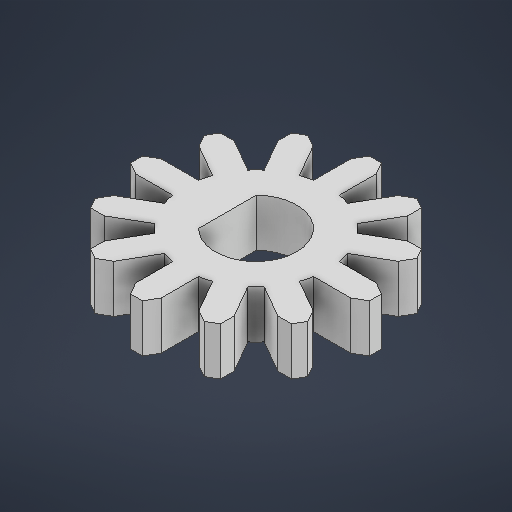
# Autodesk Inventor part: Gear
Saved by Autodesk Inventor 2026.2 (Build 302298010, 298A)
## iProperties
Created: 2026-04-14
Part Number: Gear
Material: Genérico
Document SubType Name: Modeling
Designer: pauli
Density: 1 g/cm^3
Appearance: Padrão
Author: pauli
Autodesk Inventor part; units mm, degrees
ref_plane "YZ Plane" through (0, 0, 0) normal (1, 0, 0) x (0, 1, 0)
ref_plane "XZ Plane" through (0, 0, 0) normal (0, 1, 0) x (-1, 0, 0)
ref_plane "XY Plane" through (0, 0, 0) normal (0, 0, 1) x (1, 0, 0)
sketch "Esboço1" plane through (0, 0, 0) normal (0, 1, 0) x (-1, 0, 0)
  arc A0 (1, 1.118) -> (1, -1.118) centre (0, 0) ccw construction
  line L0 (1, 1.118) -> (1, -1.118) construction
  line L1 (0, 0) -> (-1.5, 0) construction
  line L2 (1.2, -1.2042) -> (1.2, 1.2042)
  arc A1 (1.2, 1.2042) -> (1.2, -1.2042) centre (0, 0) ccw
  circle A2 centre (0, 0) radius 3
  point P0 (1, 0)
  dimension "d0" = 3
  dimension "d1" = 2.5
  dimension "d2" = 0.2
  dimension "d3" = 6
  constraints: 6 end point, 5 point on circle, 3 centre point, 2 coincident, 1 horizontal, 1 midpoint, 1 vertical, 1 other
  measures "d0" diameter of A0
  measures "d1" distance of L1.end point (1, 0)
  measures "d2" distance between parallel lines of L0 L2
  measures "d3" diameter of A2
extrude "Extrusão1" add sketch "Esboço1" along normal blind 2
sketch "Esboço2" plane through (0, 2, 0) normal (0, 1, 0) x (1, 0, 0)
  line L0 (0, 0) -> (-5, 0) construction
  line L1 (-5, 0) -> (-5, 0.25)
  line L2 (-5, 0.25) -> (-4.5, 0.5387)
  line L3 (-4.5, 0.5387) -> (-2.8873, 0.5387)
  line L4 (-5, 0) -> (-5, -0.25)
  line L5 (-5, -0.25) -> (-4.5, -0.5387)
  line L6 (-4.5, -0.5387) -> (-2.8873, -0.5387)
  line L7 (-4.3301, -2.5) -> (-4.4551, -2.2835)
  line L8 (-4.4551, -2.2835) -> (-4.1665, -1.7835)
  line L9 (-4.1665, -1.7835) -> (-2.7698, -0.9771)
  line L10 (-4.3301, -2.5) -> (-4.2051, -2.7165)
  line L11 (-4.2051, -2.7165) -> (-3.6278, -2.7165)
  line L12 (-3.6278, -2.7165) -> (-2.2311, -1.9102)
  line L13 (-2.5, -4.3301) -> (-2.7165, -4.2051)
  line L14 (-2.7165, -4.2051) -> (-2.7165, -3.6278)
  line L15 (-2.7165, -3.6278) -> (-1.9102, -2.2311)
  line L16 (-2.5, -4.3301) -> (-2.2835, -4.4551)
  line L17 (-2.2835, -4.4551) -> (-1.7835, -4.1665)
  line L18 (-1.7835, -4.1665) -> (-0.9771, -2.7698)
  line L19 (0, -5) -> (-0.25, -5)
  line L20 (-0.25, -5) -> (-0.5387, -4.5)
  line L21 (-0.5387, -4.5) -> (-0.5387, -2.8873)
  line L22 (0, -5) -> (0.25, -5)
  line L23 (0.25, -5) -> (0.5387, -4.5)
  line L24 (0.5387, -4.5) -> (0.5387, -2.8873)
  line L25 (2.5, -4.3301) -> (2.2835, -4.4551)
  line L26 (2.2835, -4.4551) -> (1.7835, -4.1665)
  line L27 (1.7835, -4.1665) -> (0.9771, -2.7698)
  line L28 (2.5, -4.3301) -> (2.7165, -4.2051)
  line L29 (2.7165, -4.2051) -> (2.7165, -3.6278)
  line L30 (2.7165, -3.6278) -> (1.9102, -2.2311)
  line L31 (4.3301, -2.5) -> (4.2051, -2.7165)
  line L32 (4.2051, -2.7165) -> (3.6278, -2.7165)
  line L33 (3.6278, -2.7165) -> (2.2311, -1.9102)
  line L34 (4.3301, -2.5) -> (4.4551, -2.2835)
  line L35 (4.4551, -2.2835) -> (4.1665, -1.7835)
  line L36 (4.1665, -1.7835) -> (2.7698, -0.9771)
  line L37 (5, 0) -> (5, -0.25)
  line L38 (5, -0.25) -> (4.5, -0.5387)
  line L39 (4.5, -0.5387) -> (2.8873, -0.5387)
  line L40 (5, 0) -> (5, 0.25)
  line L41 (5, 0.25) -> (4.5, 0.5387)
  line L42 (4.5, 0.5387) -> (2.8873, 0.5387)
  line L43 (4.3301, 2.5) -> (4.4551, 2.2835)
  line L44 (4.4551, 2.2835) -> (4.1665, 1.7835)
  line L45 (4.1665, 1.7835) -> (2.7698, 0.9771)
  line L46 (4.3301, 2.5) -> (4.2051, 2.7165)
  line L47 (4.2051, 2.7165) -> (3.6278, 2.7165)
  line L48 (3.6278, 2.7165) -> (2.2311, 1.9102)
  line L49 (2.5, 4.3301) -> (2.7165, 4.2051)
  line L50 (2.7165, 4.2051) -> (2.7165, 3.6278)
  line L51 (2.7165, 3.6278) -> (1.9102, 2.2311)
  line L52 (2.5, 4.3301) -> (2.2835, 4.4551)
  line L53 (2.2835, 4.4551) -> (1.7835, 4.1665)
  line L54 (1.7835, 4.1665) -> (0.9771, 2.7698)
  line L55 (0, 5) -> (0.25, 5)
  line L56 (0.25, 5) -> (0.5387, 4.5)
  line L57 (0.5387, 4.5) -> (0.5387, 2.8873)
  line L58 (0, 5) -> (-0.25, 5)
  line L59 (-0.25, 5) -> (-0.5387, 4.5)
  line L60 (-0.5387, 4.5) -> (-0.5387, 2.8873)
  line L61 (-2.5, 4.3301) -> (-2.2835, 4.4551)
  line L62 (-2.2835, 4.4551) -> (-1.7835, 4.1665)
  line L63 (-1.7835, 4.1665) -> (-0.9771, 2.7698)
  line L64 (-2.5, 4.3301) -> (-2.7165, 4.2051)
  line L65 (-2.7165, 4.2051) -> (-2.7165, 3.6278)
  line L66 (-2.7165, 3.6278) -> (-1.9102, 2.2311)
  line L67 (-4.3301, 2.5) -> (-4.2051, 2.7165)
  line L68 (-4.2051, 2.7165) -> (-3.6278, 2.7165)
  line L69 (-3.6278, 2.7165) -> (-2.2311, 1.9102)
  line L70 (-4.3301, 2.5) -> (-4.4551, 2.2835)
  line L71 (-4.4551, 2.2835) -> (-4.1665, 1.7835)
  line L72 (-4.1665, 1.7835) -> (-2.7698, 0.9771)
  circle A0 centre (0, 0) radius 3
  point P0 (-1.0091, -2.8252)
  point P1 (-1.9421, -2.2865)
  point P2 (-2.2865, -1.9421)
  point P3 (-2.8252, -1.0091)
  point P4 (-2.9512, -0.5387)
  point P5 (-2.9512, 0.5387)
  point P6 (-2.8252, 1.0091)
  point P7 (-2.2865, 1.9421)
  point P8 (-1.9421, 2.2865)
  point P9 (-1.0091, 2.8252)
  point P10 (-0.5387, 2.9512)
  point P11 (0.5387, 2.9512)
  point P12 (1.0091, 2.8252)
  point P13 (1.9421, 2.2865)
  point P14 (2.2865, 1.9421)
  point P15 (2.8252, 1.0091)
  point P16 (2.9512, 0.5387)
  point P17 (2.9512, -0.5387)
  point P18 (2.8252, -1.0091)
  point P19 (2.2865, -1.9421)
  point P20 (1.9421, -2.2865)
  point P21 (1.0091, -2.8252)
  point P22 (0.5387, -2.9512)
  point P23 (-0.5387, -2.9512)
  dimension "d15" = 6
  dimension "d6" = 5
  dimension "d7" = 0.25
  dimension "d9" = 60
  dimension "d10" = 0.5
  dimension "d13" = 360
  constraints: 146 end point, 3 symmetric about line, 2 horizontal, 1 coincident, 1 vertical, 159 other
  measures "d6" distance of L0.start L0.end
  measures "d7" distance of L0.end L1.end
  measures "d9" angle of L2 L1
  measures "d10" horizontal distance of L2.end L1.end
extrude "Extrusão2" add sketch "Esboço2" against normal blind 2 contours L1 L2 L3 A0 L6 L5 L4 | L72 L71 L70 L67 L68 L69 A0 | A0 L12 L11 L10 L7 L8 L9 | L66 L65 L64 L61 L62 L63 A0 | A0 L18 L17 L16 L13 L14 L15 | L60 L59 L58 L55 L56 L57 A0 | A0 L24 L23 L22 L19 L20 L21 | L54 L53 L52 L49 L50 L51 A0 | A0 L30 L29 L28 L25 L26 L27 | L48 L47 L46 L43 L44 L45 A0 | A0 L36 L35 L34 L31 L32 L33 | L42 L41 L40 L37 L38 L39 A0
